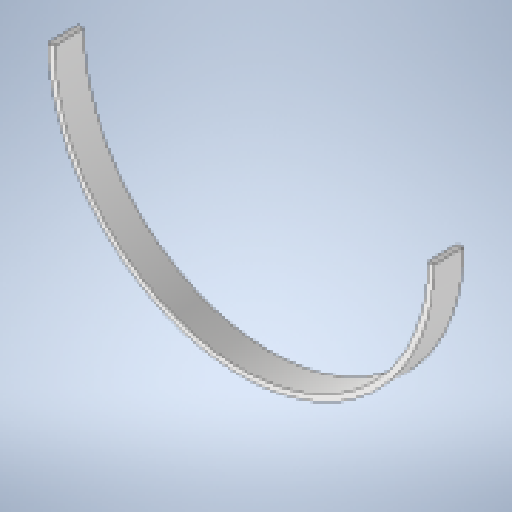
# Autodesk Inventor part: ДМФ 092 Постель НОС v2.0
Saved by Autodesk Inventor 2025 (Build 290162010, 162A)
## iProperties
Created: 2024-04-28
Part Number: ДМФ 092 Постель НОС v2.0
Material: Generic
Document SubType Name: Sheet Metal
Designer: admin
Stock Number: Постель_Нос
Density: 1 g/cm^3
Sheet Metal Rule: Default
Sheet Metal Width: 0,000 mm
Sheet Metal Length: 0,000 mm
Sheet Metal Area: 0,000 mm^2
Appearance: Default
Author: pokla
Autodesk Inventor part; units mm, degrees
note: some values were not read from the file. Chosen so that the rebuilt part matches the saved one: flange form of "Plate1".
ref_plane "YZ Plane" through (0, 0, 0) normal (1, 0, 0) x (0, 1, 0)
ref_plane "XZ Plane" through (0, 0, 0) normal (0, 1, 0) x (-1, 0, 0)
ref_plane "XY Plane" through (0, 0, 0) normal (0, 0, 1) x (1, 0, 0)
sketch "Sketch8" plane through (0, 0, 0) normal (0, 0, 1) x (1, 0, 0)
  arc A0 (-165, 0) -> (165, 0) centre (0, 0) ccw
  dimension "d46" = 330
  measures "d46" distance of A0.end A0.start
contour flange "Contour Flange1" sketch "Sketch8" thickness 6 bend radius 6 width 30 along (0, 0, 1) mid plane no both sides no wall seen from (0, -165, 0) lies toward (0, -1, 0) curves A0
bend "Bend1"
corner "Corner1"
equation "\"d47\" = Thickness"
equation "\"d48\" = BendReliefWidth"
equation "\"d49\" = BendReliefDepth"
equation "\"d50\" = MinimumRemnant"
equation "\"d51\" = TransitionRadius"
equation "\"d53\" = BendRadius"
equation "\"d55\" = CornerReliefSize"
equation "\"d56\" = GapSize"
equation "\"d57\" = JacobiRadiusSize"
equation "\"BendRadius\" = Thickness"
equation "\"BendReliefWidth\" = Thickness"
equation "\"BendReliefDepth\" = 0.5 * Thickness"
equation "\"CornerReliefSize\" = 4 * Thickness"
equation "\"MinimumRemnant\" = 2 * Thickness"
equation "\"TransitionRadius\" = BendRadius"
equation "\"JacobiRadiusSize\" = BendRadius"
equation "\"GapSize\" = Thickness"
equation "\"Thickness\" = 6"
body "Solid2"
